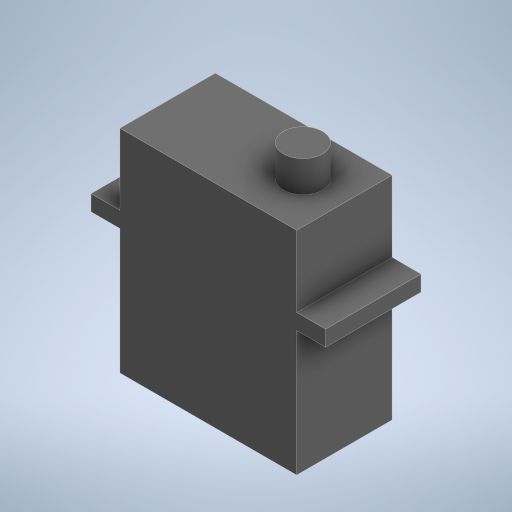
# Autodesk Inventor part: Servo_small_maketa
Saved by Autodesk Inventor 2023 (Build 270158000, 158)
## iProperties
Created: 2024-06-26
Part Number: Servo_small_maketa
Material: Generic
Document SubType Name: Modeling
Designer: Swoby
Density: 1 g/cm^3
Appearance: Default
Author: Swoby
Autodesk Inventor part; units mm, degrees
ref_plane "YZ Plane" through (0, 0, 0) normal (1, 0, 0) x (0, 1, 0)
ref_plane "XZ Plane" through (0, 0, 0) normal (0, 1, 0) x (-1, 0, 0)
ref_plane "XY Plane" through (0, 0, 0) normal (0, 0, 1) x (1, 0, 0)
sketch "Sketch1" plane through (0, 0, 0) normal (0, 1, 0) x (-1, 0, 0)
  line L0 (-11.3, 6.1) -> (11.3, 6.1)
  line L1 (11.3, 6.1) -> (11.3, -6.1)
  line L2 (11.3, -6.1) -> (-11.3, -6.1)
  line L3 (-11.3, -6.1) -> (-11.3, 6.1)
  line L4 (-11.3, 6.1) -> (11.3, -6.1) construction
  line L5 (11.3, 6.1) -> (-11.3, -6.1) construction
  point P0 (0, 0)
  dimension "d0" = 22.6
  dimension "d1" = 12.2
  constraints: 12 end point, 2 midpoint, 2 parallel, 1 horizontal, 1 perpendicular
  measures "d0" distance of L1.end L2.end
  measures "d1" distance of L0.end L1.end
extrude "Extrusion1" add sketch "Sketch1" along normal blind 27.1
ref_plane "Work Plane1" through (0, 16, 0) normal (0, -1, 0) x (1, 0, 0)
sketch "Sketch2" plane through (0, 16, 0) normal (0, -1, 0) x (1, 0, 0)
  line L0 (-11.3, 6.1) -> (11.3, 6.1) projected
  line L1 (11.3, 6.1) -> (15, 6.1)
  line L2 (15, 6.1) -> (15, -6.1)
  line L3 (15, -6.1) -> (11.3, -6.1)
  line L4 (11.3, -6.1) -> (11.3, 6.1)
  line L5 (-11.3, -6.1) -> (-11.3, 6.1) projected
  line L6 (-11.3, 6.1) -> (-15, 6.1)
  line L7 (-15, 6.1) -> (-15, -6.1)
  line L8 (-15, -6.1) -> (-11.3, -6.1)
  line L9 (-11.3, -6.1) -> (-11.3, 6.1)
  line L10 (11.3, -6.1) -> (-11.3, -6.1) projected
  point P0 (0, 0)
  dimension "d5" = 30
  dimension "d6" = 22.6
  dimension "d7" = 3.7
  constraints: 16 end point, 4 parallel, 2 horizontal, 2 perpendicular, 1 point on line
  measures "d5" distance between parallel lines of L7 L2
  measures "d6" distance of L3.end L5.start
  measures "d7" distance of L2.end L3.end
extrude "Extrusion2" add sketch "Sketch2" against normal blind 2 contours L5 L8 L7 L6 | L1 L2 L3 L4
sketch "Sketch3" plane through (0, 27.1, 0) normal (0, 1, 0) x (1, 0, 0)
  circle A0 centre (6, 0) radius 2.5
  line L0 (15, -6.1) -> (15, 6.1) projected
  point P0 (0, 0)
  dimension "d10" = 5
  dimension "d11" = 9
  constraints: 1 centre point
  measures "d10" diameter of A0
  measures "d11" distance from line of A0.centre L0
extrude "Extrusion3" add sketch "Sketch3" along normal blind 4
equation "\"d7\" = -0.5 * d6 + 0.5 * d5"
body "Solid1"
